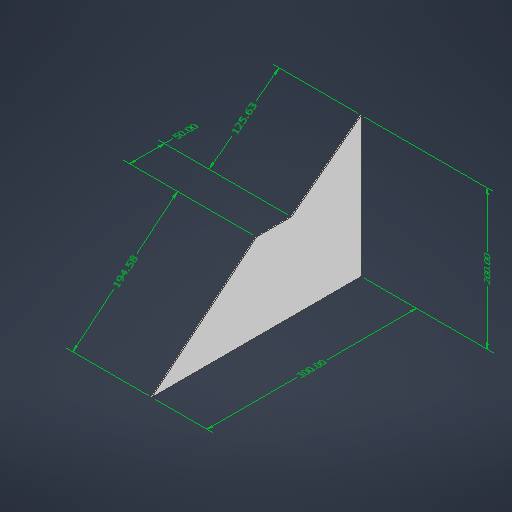
# Autodesk Inventor part: parte lateral
Saved by Autodesk Inventor 2027 (Build 310192060, 192F)
## iProperties
Created: 2026-09-04
Part Number: parte lateral
Material: Genérico
Document SubType Name: Modeling
Designer: Leandro
Density: 1 g/cm^3
Appearance: Valor por defecto
Author: Leandro
Autodesk Inventor part; units mm, degrees
ref_plane "YZ Plane" through (0, 0, 0) normal (1, 0, 0) x (0, 1, 0)
ref_plane "XZ Plane" through (0, 0, 0) normal (0, 1, 0) x (-1, 0, 0)
ref_plane "XY Plane" through (0, 0, 0) normal (0, 0, 1) x (1, 0, 0)
sketch "Boceto1" plane through (0, 0, 0) normal (1, 0, 0) x (0, 1, 0)
  line L0 (1.2642, 8.9824) -> (1.2642, -291.0176)
  line L1 (1.2642, -291.0176) -> (201.2642, -291.0176)
  line L2 (1.2642, 8.9824) -> (125.2111, -141.0176)
  line L3 (125.2111, -141.0176) -> (125.2111, -191.0176)
  line L4 (125.2111, -191.0176) -> (201.2642, -291.0176)
  point P0 (0, 0)
  dimension "d0" = 300
  dimension "d1" = 200
  dimension "d4" = 50
  constraints: 10 end point, 2 vertical, 1 perpendicular
  measures "d0" distance of L0.start L0.end
  measures "d1" distance of L0.end L1.end
  measures "d4" distance of L2.end L3.end
extrude "Extrusión1" add sketch "Boceto1" along normal mid plane 1.5
